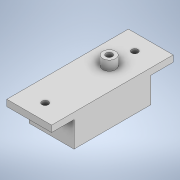
# Autodesk Inventor part: servo_sub
Saved by Autodesk Inventor 2020.1 (Build 241239000, 239)
## iProperties
Created: 2022-04-03
Part Number: servo_sub
Material: Generic
Document SubType Name: Modeling
Designer: OEM
Density: 1 g/cm^3
Appearance: Default
Author: OEM
Autodesk Inventor part; units mm, degrees
ref_plane "YZ Plane" through (0, 0, 0) normal (1, 0, 0) x (0, 1, 0)
ref_plane "XZ Plane" through (0, 0, 0) normal (0, 1, 0) x (-1, 0, 0)
ref_plane "XY Plane" through (0, 0, 0) normal (0, 0, 1) x (1, 0, 0)
sketch "Sketch1" plane through (0, 0, 0) normal (0, 1, 0) x (-1, 0, 0)
  line L0 (7, 12) -> (-7, 12)
  line L1 (-7, 12) -> (-7, -12)
  line L2 (-7, -12) -> (7, -12)
  line L3 (7, -12) -> (7, 12)
  line L4 (7, 12) -> (-7, -12) construction
  line L5 (-7, 12) -> (7, -12) construction
  circle A0 centre (0, -14) radius 1
  circle A1 centre (0, -6) radius 1
  circle A2 centre (0, 14) radius 1
  line L6 (7, 12) -> (7, 19)
  line L7 (7, 19) -> (-7, 19)
  line L8 (-7, 19) -> (-7, 12)
  line L9 (18, 0) -> (-22, 0) construction
  line L10 (7, -12) -> (7, -19)
  line L11 (7, -19) -> (-7, -19)
  line L12 (-7, -19) -> (-7, -12)
  circle A3 centre (0, -6) radius 2
  point P0 (0, 0)
  point P1 (0, 0)
  point P2 (0, 0)
  point P3 (14, -24)
  point P4 (0, 0)
  point P5 (7, 0)
  point P6 (-7, 24)
  dimension "d0" = 14
  dimension "d1" = 24
  dimension "d2" = 2
  dimension "d3" = 2
  dimension "d4" = 6
  dimension "d5" = 2
  dimension "d6" = 7
  dimension "d11" = 4
  constraints: 26 end point, 4 centre point, 4 midpoint, 3 perpendicular, 2 horizontal, 2 parallel, 2 point on line, 2 symmetric about line, 1 coincident, 1 vertical, 1 other
  measures "d0" distance of L2.start L2.end
  measures "d1" distance of L2.end L4.start
  measures "d2" diameter of A0
  measures "d3" distance from line of L2 A0.centre
  measures "d4" distance from line of L2 A1.centre
  measures "d5" diameter of A1
  measures "d6" distance between parallel lines of L7 L0
  measures "d11" diameter of A3
extrude "Extrusion1" add sketch "Sketch1" against normal blind 10 contours L3 L2 L1 L0 | A1 | A3
extrude "Extrusion2" add sketch "Sketch1" against normal blind 2 contours L0 L8 L7 L6 | L10 L11 L12 L2
extrude "Extrusion3" add sketch "Sketch1" along normal blind 3 contours A3
body "Solid1"
